Head v8 (Autodesk Fusion 360 design; units mm, degrees)
Autodesk Fusion 360 part; units mm, degrees
note: some values were not read from the file. Set by a fixed rule: which sketch regions a step uses.
sketch "RobotSatan_Outline_2" plane through (0, 0, 0) normal (0, 1, 0) x (1, 0, 0)
  spline S0 degree 3 poles (10.235, 114.5284) (8.6125, 114.5284) (7.297, 113.2125) (7.297, 111.5894) knots 0 0 0 0 1 1 1 1
  spline S1 degree 3 poles (27.2951, 30.5045) (28.9523, 30.5045) (29.7315, 29.3352) (29.7315, 27.8928) knots 0 0 0 0 1 1 1 1
  spline S2 degree 3 poles (10.235, 70.9521) (11.1129, 70.9036) (11.6031, 70.3892) (11.5794, 69.7582) knots 0 0 0 0 1 1 1 1
  spline S3 degree 3 poles (52.0987, 28.374) (53.7202, 28.4279) (55.0356, 29.69) (55.0356, 31.3131) knots 0 0 0 0 1 1 1 1
  spline S4 degree 3 poles (18.5903, 27.8928) (18.5903, 29.3352) (19.3689, 30.5045) (21.0261, 30.5045) knots 0 0 0 0 1 1 1 1
  line L0 (50.7482, 117.3562) -> (50.7482, 115.7102)
  line L1 (7.297, 73.8917) -> (7.297, 82.2427) construction
  line L2 (55.0356, 111.5894) -> (55.0356, 108.6938)
  spline S5 degree 3 poles (11.5794, 115.708) (11.6016, 114.9323) (11.1123, 114.6075) (10.235, 114.5284) knots 0 0 0 0 1 1 1 1
  spline S6 degree 3 poles (11.5794, 19.4245) (11.5794, 17.8014) (12.8944, 16.4854) (14.5168, 16.4854) knots 0 0 0 0 1 1 1 1
  line L3 (27.2951, 23.1855) -> (21.0261, 23.1855)
  spline S7 degree 3 poles (50.7482, 104.5729) (50.749, 105.0607) (51.0594, 105.7079) (52.0987, 105.7553) knots 0 0 0 0 1 1 1 1
  line L4 (29.7315, 27.8928) -> (29.7315, 25.7971)
  line L5 (50.7482, 19.4245) -> (50.7482, 27.1735)
  spline S8 degree 3 poles (50.7482, 117.3562) (50.7482, 118.9793) (49.4332, 120.2947) (47.8108, 120.2947) knots 0 0 0 0 1 1 1 1
  spline S9 degree 3 poles (14.5168, 120.2947) (12.8944, 120.2947) (11.5794, 118.9793) (11.5794, 117.3562) knots 0 0 0 0 1 1 1 1
  line L6 (14.5168, 16.4854) -> (22.8385, 16.4854)
  line L7 (22.3658, 46.6652) -> (19.6342, 46.6652)
  line L8 (28.812, 14.3765) -> (33.4439, 14.3765)
  line L9 (18.5903, 27.8928) -> (18.5903, 25.7971)
  spline S10 degree 3 poles (21.0261, 23.1855) (19.3689, 23.1855) (18.6453, 24.3555) (18.5903, 25.7971) knots 0 0 0 0 1 1 1 1
  spline S11 degree 3 poles (10.235, 28.374) (10.7285, 28.3793) (11.6383, 28.108) (11.5794, 27.2452) knots 0 0 0 0 1 1 1 1
  spline S12 degree 3 poles (11.5794, 43.7193) (11.5828, 43.2312) (11.1144, 42.5873) (10.235, 42.6031) knots 0 0 0 0 1 1 1 1
  spline S13 degree 3 poles (52.0987, 114.5284) (51.2509, 114.5136) (50.7594, 115.2803) (50.7482, 115.7102) knots 0 0 0 0 1 1 1 1
  line L10 (14.5168, 100.5358) -> (47.8108, 100.5358)
  spline S14 degree 3 poles (47.8108, 16.4854) (49.4323, 16.5393) (50.7482, 17.8014) (50.7482, 19.4245) knots 0 0 0 0 1 1 1 1
  line L11 (27.1821, 15.8565) -> (27.1821, 15.6906)
  line L12 (27.2951, 30.5045) -> (21.0261, 30.5045)
  line L13 (61.8594, 0.1406) -> (0.1406, 0.1406)
  line L14 (14.5168, 120.2947) -> (47.8108, 120.2947)
  line L15 (21.0261, 30.5045) -> (27.2951, 30.5045)
  line L16 (21.0261, 23.1855) -> (27.2951, 23.1855)
  spline S15 degree 3 poles (52.0987, 105.7553) (53.7211, 105.7553) (55.0356, 107.0707) (55.0356, 108.6938) knots 0 0 0 0 1 1 1 1
  line L17 (33.4439, 17.1706) -> (28.812, 17.1706)
  spline S16 degree 3 poles (29.7315, 25.7971) (29.7315, 24.3547) (28.9523, 23.1855) (27.2951, 23.1855) knots 0 0 0 0 1 1 1 1
  line L18 (18.5903, 25.7971) -> (18.5903, 27.8928)
  spline S17 degree 3 poles (38.2753, 14.9635) (38.2769, 16.2773) (39.0062, 16.4966) (39.4957, 16.4854) knots 0 0 0 0 1 1 1 1
  spline S18 degree 3 poles (10.235, 42.6031) (8.6125, 42.6031) (7.297, 41.2877) (7.297, 39.6646) knots 0 0 0 0 1 1 1 1
  spline S19 degree 3 poles (10.235, 105.7553) (11.1266, 105.7379) (11.5873, 104.8858) (11.5794, 104.5647) knots 0 0 0 0 1 1 1 1
  line L19 (42.3658, 46.6652) -> (39.6342, 46.6652)
  spline S20 degree 3 poles (35.3373, 12.025) (36.9598, 12.025) (38.2753, 13.3404) (38.2753, 14.9635) knots 0 0 0 0 1 1 1 1
  line L20 (47.8108, 120.2947) -> (14.5168, 120.2947)
  line L21 (39.4957, 16.4854) -> (47.8108, 16.4854)
  line L22 (35.0744, 15.8565) -> (35.0744, 15.6906)
  line L23 (33.4439, 14.3765) -> (28.812, 14.3765)
  line L24 (29.7315, 25.7971) -> (29.7315, 27.8928)
  line L25 (35.0744, 15.6906) -> (35.0744, 15.8565)
  line L26 (7.297, 108.6938) -> (7.297, 111.5894)
  line L27 (11.5794, 115.708) -> (11.5794, 117.3562)
  spline S21 degree 3 poles (27.1821, 15.8565) (27.1821, 16.5823) (27.9117, 17.1706) (28.812, 17.1706) knots 0 0 0 0 1 1 1 1
  line L28 (11.5794, 104.5647) -> (11.5794, 103.4749)
  spline S22 degree 3 poles (50.7482, 69.7345) (50.7292, 70.4446) (51.1934, 70.9205) (52.0987, 70.9521) knots 0 0 0 0 1 1 1 1
  line L29 (7.297, 111.5894) -> (7.297, 108.6938)
  spline S23 degree 3 poles (7.297, 108.6938) (7.3508, 107.0716) (8.6125, 105.7553) (10.235, 105.7553) knots 0 0 0 0 1 1 1 1
  line L30 (11.5794, 117.3562) -> (11.5794, 115.708)
  spline S24 degree 3 poles (55.0356, 111.5894) (55.0356, 113.2125) (53.7211, 114.5284) (52.0987, 114.5284) knots 0 0 0 0 1 1 1 1
  line L31 (50.7482, 104.5729) -> (50.7482, 103.4749)
  line L32 (50.7482, 103.4749) -> (50.7482, 104.5729)
  line L33 (35.3373, 12.025) -> (26.9903, 12.025)
  line L34 (50.7482, 115.7102) -> (50.7482, 117.3562)
  line L35 (11.5794, 69.7582) -> (11.5794, 43.7193)
  line L36 (7.297, 39.6646) -> (7.297, 31.3131)
  line L37 (11.5794, 27.2452) -> (11.5794, 19.4245)
  line L38 (7.297, 31.3131) -> (7.297, 39.6646)
  line L39 (55.0356, 108.6938) -> (55.0356, 111.5894)
  line L40 (50.7482, 27.1735) -> (50.7482, 19.4245)
  line L41 (47.8108, 100.5358) -> (14.5168, 100.5358)
  line L42 (55.0356, 82.2427) -> (55.0356, 73.8917)
  spline S25 degree 3 poles (47.8108, 100.5358) (49.4323, 100.5897) (50.7482, 101.8518) (50.7482, 103.4749) knots 0 0 0 0 1 1 1 1
  line L43 (50.7482, 43.786) -> (50.7482, 69.7345)
  line L44 (28.812, 17.1706) -> (33.4439, 17.1706)
  line L45 (27.1821, 15.6906) -> (27.1821, 15.8565)
  line L46 (11.5794, 103.4749) -> (11.5794, 104.5647)
  line L47 (50.7482, 69.7345) -> (50.7482, 43.786)
  spline S26 degree 3 poles (24.0523, 14.9635) (24.1061, 13.3413) (25.3678, 12.025) (26.9903, 12.025) knots 0 0 0 0 1 1 1 1
  line L48 (11.5794, 43.7193) -> (11.5794, 69.7582)
  spline S27 degree 3 poles (22.8385, 16.4854) (23.3022, 16.5043) (24.0076, 16.1123) (24.0523, 14.9635) knots 0 0 0 0 1 1 1 1
  spline S28 degree 3 poles (35.0744, 15.6906) (35.0744, 14.9648) (34.3442, 14.3765) (33.4439, 14.3765) knots 0 0 0 0 1 1 1 1
  line L49 (26.9903, 12.025) -> (35.3373, 12.025)
  line L50 (55.0356, 73.8917) -> (55.0356, 82.2427)
  line L51 (11.5794, 19.4245) -> (11.5794, 27.2452)
  spline S29 degree 3 poles (7.297, 31.3131) (7.297, 29.69) (8.6125, 28.374) (10.235, 28.374) knots 0 0 0 0 1 1 1 1
  line L52 (32.3658, 46.6652) -> (29.6342, 46.6652)
  line L53 (0.1406, 0.1406) -> (0.1406, 121.8594)
  line L54 (47.8108, 16.4854) -> (39.4957, 16.4854)
  spline S30 degree 3 poles (52.0987, 70.9521) (53.7202, 71.006) (55.0356, 72.2686) (55.0356, 73.8917) knots 0 0 0 0 1 1 1 1
  spline S31 degree 3 poles (33.4439, 17.1706) (34.3442, 17.1706) (35.0744, 16.5823) (35.0744, 15.8565) knots 0 0 0 0 1 1 1 1
  spline S32 degree 3 poles (11.5794, 103.4749) (11.5794, 101.8518) (12.8944, 100.5358) (14.5168, 100.5358) knots 0 0 0 0 1 1 1 1
  line L55 (22.8385, 16.4854) -> (14.5168, 16.4854)
  spline S33 degree 3 poles (55.0356, 39.6646) (55.0356, 41.2877) (53.7211, 42.6031) (52.0987, 42.6031) knots 0 0 0 0 1 1 1 1
  spline S34 degree 3 poles (50.7482, 27.1735) (50.7463, 28.0057) (51.624, 28.3964) (52.0987, 28.374) knots 0 0 0 0 1 1 1 1
  spline S35 degree 3 poles (7.297, 73.8917) (7.297, 72.2686) (8.6125, 70.9521) (10.235, 70.9521) knots 0 0 0 0 1 1 1 1
  line L56 (55.0356, 31.3131) -> (55.0356, 39.6646)
  spline S36 degree 3 poles (28.812, 14.3765) (27.9117, 14.3765) (27.212, 14.9652) (27.1821, 15.6906) knots 0 0 0 0 1 1 1 1
  spline S37 degree 3 poles (52.0987, 42.6031) (51.0209, 42.5992) (50.737, 43.4395) (50.7482, 43.786) knots 0 0 0 0 1 1 1 1
  line L57 (55.0356, 39.6646) -> (55.0356, 31.3131)
  line L58 (61.8594, 121.8594) -> (61.8594, 0.1406)
  line L59 (0.1406, 121.8594) -> (61.8594, 121.8594)
  spline S38 degree 3 poles (32.4655, 143.4) (23.7353, 143.4503) (14.7543, 139.3652) (8.8222, 129.236) knots 0 0 0 0 1 1 1 1
  spline S39 degree 3 poles (-8.0125, 95.4824) (-4.6273, 94.9818) (-1.6894, 95.1386) (0.7276, 95.7376) knots 0 0 0 0 1 1 1 1
  spline S40 degree 3 poles (3.7466, 109.0725) (3.7475, 109.0731) (3.7485, 109.0742) (3.7494, 109.0748) knots 0 0 0 0 1 1 1 1
  spline S41 degree 3 poles (61.918, 105.4461) (62.3441, 106.388) (61.5048, 105.6412) (58.7789, 105.6098) knots 0 0 0 0 1 1 1 1
  spline S42 degree 3 poles (8.8222, 129.236) (6.0519, 124.5056) (6.9924, 118.038) (5.4372, 112.5441) knots 0 0 0 0 1 1 1 1
  spline S43 degree 3 poles (53.6696, 133.8916) (48.6461, 139.6563) (40.6666, 143.3529) (32.4655, 143.4001) knots 0 0 0 0 1 1 1 1
  spline S44 degree 3 poles (24.2524, 66.9983) (22.9484, 63.6454) (80.6805, 92.1452) (55.5432, 101.6168) knots 0 0 0 0 1 1 1 1
  spline S45 degree 3 poles (3.5267, 109.1834) (2.9555, 109.457) (1.8977, 109.5026) (0.8037, 109.1696) knots 0 0 0 0 1 1 1 1
  spline S46 degree 3 poles (5.4372, 112.5441) (5.2254, 110.4206) (4.1381, 109.3015) (3.7494, 109.0747) knots 0 0 0 0 1 1 1 1
  spline S47 degree 3 poles (3.6435, 109.1249) (3.6041, 109.1443) (3.5666, 109.1642) (3.5267, 109.1834) knots 0 0 0 0 1 1 1 1
  spline S48 degree 3 poles (3.7615, 109.0654) (3.7566, 109.0679) (3.7515, 109.0701) (3.7466, 109.0725) knots 0 0 0 0 1 1 1 1
  line L60 (32.4655, 143.4) -> (32.4655, 143.4001)
  spline S49 degree 3 poles (0.7276, 95.7376) (-16.7215, 76.039) (36.655, 80.3237) (24.2524, 66.9983) knots 0 0 0 0 1 1 1 1
  spline S50 degree 3 poles (58.7789, 105.6098) (59.7712, 116.9489) (58.3276, 128.5464) (53.6696, 133.8916) knots 0 0 0 0 1 1 1 1
  spline S51 degree 3 poles (55.5432, 101.6168) (57.9111, 102.4984) (60.0987, 103.7515) (61.918, 105.4461) knots 0 0 0 0 1 1 1 1
  spline S52 degree 3 poles (3.6562, 109.1475) (3.6494, 109.1382) (3.6488, 109.1332) (3.6435, 109.1249) knots 0 0 0 0 1 1 1 1
  line L61 (32.4655, 143.4001) -> (32.4655, 143.4)
  spline S53 degree 3 poles (3.7494, 109.0748) (3.7206, 109.096) (3.6836, 109.1282) (3.6562, 109.1475) knots 0 0 0 0 1 1 1 1
  spline S54 degree 3 poles (3.7494, 109.0747) (3.7531, 109.0719) (3.7577, 109.0682) (3.7615, 109.0654) knots 0 0 0 0 1 1 1 1
  spline S55 degree 3 poles (0.8037, 109.1696) (-12.8378, 101.9111) (5.3858, 99.0443) (-8.0125, 95.4824) knots 0 0 0 0 1 1 1 1
  line L62 (7.147, 111.5894) -> (7.147, 108.6913)
  spline S56 degree 3 poles (7.147, 108.6913) (7.147, 108.6905) (7.1471, 108.6897) (7.1471, 108.6888) (7.2034, 106.9921) (8.5306, 105.6061) (10.2335, 105.6053) knots -0.000511 -0.000511 -0.000511 -0.000511 0 0 0 0.999702 0.999702 0.999702 0.999702
  spline S57 degree 3 poles (10.2335, 105.6053) (10.7603, 105.5944) (11.1167, 105.257) (11.2985, 104.9443) (11.3914, 104.7845) (11.4309, 104.6263) (11.4294, 104.5684) (11.4294, 104.5677) (11.4294, 104.5671) (11.4294, 104.5665) knots 0.000588 0.000588 0.000588 0.000588 0.661876 0.661876 0.661876 1 1 1 1.001915 1.001915 1.001915 1.001915
  line L63 (11.4294, 103.4749) -> (11.4294, 104.5665)
  spline S58 degree 3 poles (11.4294, 103.4749) (11.4294, 101.7707) (12.8133, 100.3858) (14.5168, 100.3858) knots 0 0 0 0 1 1 1 1
  line L64 (14.5168, 100.3858) -> (47.8133, 100.3858)
  spline S59 degree 3 poles (47.8133, 100.3858) (47.8141, 100.3859) (47.8149, 100.3859) (47.8158, 100.3859) (49.5123, 100.4423) (50.8982, 101.7707) (50.8982, 103.4749) knots -0.000512 -0.000512 -0.000512 -0.000512 0 0 0 1 1 1 1
  line L65 (50.8982, 103.4749) -> (50.8982, 104.5727)
  spline S60 degree 3 poles (50.8982, 104.5727) (50.8988, 104.9717) (51.1034, 105.4899) (51.9385, 105.5917) (51.9905, 105.598) (52.045, 105.6026) (52.1022, 105.6053) knots 0 0 0 0 0.940352 0.940352 0.940352 0.998867 0.998867 0.998867 0.998867
  spline S61 degree 3 poles (52.1022, 105.6053) (53.8041, 105.6072) (55.1856, 106.9909) (55.1856, 108.6938) knots 0.000688 0.000688 0.000688 0.000688 1 1 1 1
  line L66 (55.1856, 108.6938) -> (55.1856, 111.5894)
  spline S62 degree 3 poles (55.1856, 111.5894) (55.1856, 113.2935) (53.8022, 114.6784) (52.0987, 114.6784) (52.0982, 114.6784) (52.0978, 114.6784) (52.0974, 114.6784) knots 0 0 0 0 1 1 1 1.00027 1.00027 1.00027 1.00027
  spline S63 degree 3 poles (52.0974, 114.6784) (52.0969, 114.6784) (52.0965, 114.6784) (52.096, 114.6784) (51.4522, 114.6671) (51.039, 115.1733) (50.9284, 115.5426) (50.9093, 115.6064) (50.8996, 115.665) (50.8982, 115.7123) knots -0.000517 -0.000517 -0.000517 -0.000517 0 0 0 0.851167 0.851167 0.851167 0.998126 0.998126 0.998126 0.998126
  line L67 (50.8982, 115.7123) -> (50.8982, 117.3562)
  spline S64 degree 3 poles (50.8982, 117.3562) (50.8982, 119.0603) (49.5143, 120.4447) (47.8108, 120.4447) knots 0 0 0 0 1 1 1 1
  line L68 (47.8108, 120.4447) -> (14.5168, 120.4447)
  spline S65 degree 3 poles (14.5168, 120.4447) (12.8133, 120.4447) (11.4294, 119.0603) (11.4294, 117.3562) knots 0 0 0 0 1 1 1 1
  line L69 (11.4294, 117.3562) -> (11.4294, 115.7059)
  spline S66 degree 3 poles (11.4294, 115.7059) (11.4294, 115.7052) (11.4294, 115.7045) (11.4295, 115.7037) (11.4442, 115.1885) (11.2516, 114.9477) (10.82, 114.7957) (10.6572, 114.7384) (10.4586, 114.6996) (10.2281, 114.6784) knots -0.000923 -0.000923 -0.000923 -0.000923 0 0 0 0.724154 0.724154 0.724154 0.997406 0.997406 0.997406 0.997406
  spline S67 degree 3 poles (10.2281, 114.6784) (8.5277, 114.6747) (7.147, 113.2913) (7.147, 111.5894) knots 0.001348 0.001348 0.001348 0.001348 1 1 1 1
  line L70 (6.147, 108.6747) -> (6.147, 111.5894)
  spline S68 degree 3 poles (10.1748, 115.678) (8.283, 115.6506) (6.6845, 114.3247) (6.2588, 112.5418) (6.1856, 112.2353) (6.147, 111.9157) (6.147, 111.5894) knots 0.008942 0.008942 0.008942 0.008942 0.854617 0.854617 0.854617 1 1 1 1
  spline S69 degree 3 poles (10.4294, 115.7213) (10.3703, 115.7058) (10.2833, 115.6894) (10.1748, 115.678) knots 0.796356 0.796356 0.796356 0.796356 0.976812 0.976812 0.976812 0.976812
  line L71 (10.4294, 115.7213) -> (10.4294, 117.3562)
  spline S70 degree 3 poles (14.5168, 121.4447) (12.6021, 121.4447) (10.9764, 120.1145) (10.5432, 118.3172) (10.4687, 118.0081) (10.4294, 117.6855) (10.4294, 117.3562) knots 0 0 0 0 0.85324 0.85324 0.85324 1 1 1 1
  line L72 (14.5168, 121.4447) -> (47.8108, 121.4447)
  spline S71 degree 3 poles (51.8982, 117.3562) (51.8982, 119.2711) (50.5687, 120.8973) (48.7717, 121.3308) (48.4626, 121.4054) (48.1401, 121.4447) (47.8108, 121.4447) knots 0 0 0 0 0.853239 0.853239 0.853239 1 1 1 1
  line L73 (51.8982, 115.806) -> (51.8982, 117.3562)
  spline S72 degree 3 poles (52.0886, 115.6784) (52.0852, 115.6784) (52.0819, 115.6783) (52.0785, 115.6783) (52.0071, 115.677) (51.9994, 115.6875) (51.9497, 115.738) (51.9295, 115.7586) (51.9098, 115.7856) (51.8982, 115.806) knots -0.003967 -0.003967 -0.003967 -0.003967 0 0 0 0.485877 0.485877 0.485877 0.683858 0.683858 0.683858 0.683858
  spline S73 degree 3 poles (56.1856, 111.5894) (56.1856, 113.504) (54.8569, 115.1307) (53.0598, 115.5645) (52.7507, 115.6391) (52.4281, 115.6784) (52.0987, 115.6784) (52.0953, 115.6784) (52.092, 115.6784) (52.0886, 115.6784) knots 0 0 0 0 0.853226 0.853226 0.853226 1 1 1 1.002073 1.002073 1.002073 1.002073
  line L74 (56.1856, 111.5894) -> (56.1856, 108.6938)
  spline S74 degree 3 poles (52.1309, 104.6054) (54.03, 104.6202) (55.6386, 105.9437) (56.0708, 107.7285) (56.1459, 108.0389) (56.1856, 108.3629) (56.1856, 108.6938) knots 0.004787 0.004787 0.004787 0.004787 0.852555 0.852555 0.852555 1 1 1 1
  spline S75 degree 3 poles (51.8982, 104.5603) (51.9279, 104.5736) (51.9958, 104.5973) (52.1309, 104.6054) knots 0.740647 0.740647 0.740647 0.740647 0.987986 0.987986 0.987986 0.987986
  line L75 (51.8982, 104.5603) -> (51.8982, 103.4749)
  spline S76 degree 3 poles (47.8299, 99.3858) (47.8362, 99.386) (47.8426, 99.3863) (47.849, 99.3865) (49.5971, 99.4445) (51.1264, 100.5496) (51.6797, 102.1591) (51.8217, 102.5721) (51.8982, 103.0166) (51.8982, 103.4749) knots -0.003923 -0.003923 -0.003923 -0.003923 0 0 0 0.795824 0.795824 0.795824 1 1 1 1
  line L76 (47.8299, 99.3858) -> (14.5168, 99.3858)
  spline S77 degree 3 poles (10.4294, 103.4749) (10.4294, 101.5585) (11.7608, 99.9309) (13.56, 99.4987) (13.8678, 99.4248) (14.189, 99.3858) (14.5168, 99.3858) knots 0 0 0 0 0.853916 0.853916 0.853916 1 1 1 1
  line L77 (10.4294, 104.4494) -> (10.4294, 103.4749)
  spline S78 degree 3 poles (10.2185, 104.6053) (10.2902, 104.6022) (10.3098, 104.5874) (10.3672, 104.529) (10.3908, 104.505) (10.4139, 104.4747) (10.4294, 104.4494) knots 0.01242 0.01242 0.01242 0.01242 0.459325 0.459325 0.459325 0.642978 0.642978 0.642978 0.642978
  spline S79 degree 3 poles (6.147, 108.6747) (6.1472, 108.6684) (6.1474, 108.662) (6.1476, 108.6557) (6.2056, 106.9088) (7.308, 105.3803) (8.9151, 104.8253) (9.3242, 104.6841) (9.7645, 104.6071) (10.2185, 104.6053) knots -0.003918 -0.003918 -0.003918 -0.003918 0 0 0 0.795118 0.795118 0.795118 0.997552 0.997552 0.997552 0.997552
  line L78 (10.4294, 115.7213) -> (51.8982, 115.806)
  line L79 (52.1309, 104.6054) -> (10.2185, 104.6053)
  dimension "d3" = 0.15
  dimension "d4" = 1.15
  measures "d3" distance of L29
  measures "d4" distance of L26
extrude "Extrude1" add sketch "RobotSatan_Outline_2" along normal blind 3 contours S0 L0 L2 S5 S7 S13 S15 S19 L26 L27 L29 S23 L30 S24 L34 L39 L78 L79 | S0 S5 S19 L26 L27 L29 S23 L30 L62 S56 S57 L69 S66 S67 L78 L79 | L0 S8 S9 L14 L20 L27 L30 L34 L67 S64 L68 S65 L69 L78 | L0 S8 S9 L14 L20 L27 L30 L34 L78 | L67 S64 L68 S65 L69 L71 S70 L72 S71 L73 L78 | L62 S56 S57 L69 S66 S67 L70 S68 S69 S79 L78 L79 | L0 L2 S7 S13 S15 S24 L34 L39 S60 S61 L66 S62 S63 L67 L78 L79 | S7 L10 S19 L28 L31 L32 L41 S25 L46 S32 L79 | S7 L10 S19 L28 L31 L32 L41 S25 L46 S32 S57 L63 S58 L64 S59 L65 S60 L79 | S60 S61 L66 S62 S63 L67 S72 S73 L74 S74 L78 L79 | S57 L63 S58 L64 S59 L65 S60 S75 L75 S76 L76 S77 L77 S78 L79 | L53 L58 L59 S39 S41 S42 S44 S45 S46 S47 S49 S50 S51 S52 S53 S55 | L53 S49 | L53 S39 S55 | L59 S38 S42 S43 S50 makes body 1
extrude "Extrude2" add sketch "RobotSatan_Outline_2" against normal blind 5 separate body contours L62 S56 S57 L69 S66 S67 L70 S68 S69 S79 L78 L79 | S60 S61 L66 S62 S63 L67 S72 S73 L74 S74 L78 L79 makes body 2 at (6.2362, -2.8704, -107.9159) makes body 3 at (54.3636, -2.2222, -114.992)
extrude "Extrude3" cut sketch "RobotSatan_Outline_2" along normal through all contours S0 L0 L2 S5 S7 S13 S15 S19 L26 L27 L29 S23 L30 S24 L34 L39 L78 L79 bodies 1
sketch "Sketch3" plane through (0, 0, 0) normal (0, -1, 0) x (1, 0, 0)
  line L0 (11.5781, -104.6053) -> (50.7487, -104.6054)
  spline S0 degree 3 poles (50.7487, -104.6054) (50.763, -105.089) (51.0823, -105.7089) (52.0987, -105.7553) knots 0.022041 0.022041 0.022041 0.022041 1 1 1 1
  spline S1 degree 3 poles (52.0987, -105.7553) (53.7211, -105.7553) (55.0356, -107.0707) (55.0356, -108.6938) knots 0 0 0 0 1 1 1 1
  line L1 (55.0356, -108.6938) -> (55.0356, -111.5894)
  spline S2 degree 3 poles (55.0356, -111.5894) (55.0356, -113.2125) (53.7211, -114.5284) (52.0987, -114.5284) knots 0 0 0 0 1 1 1 1
  spline S3 degree 3 poles (52.0987, -114.5284) (51.2509, -114.5136) (50.7594, -115.2803) (50.7482, -115.7102) knots 0 0 0 0 1 1 1 1
  line L2 (50.7482, -115.7102) -> (50.7482, -115.8036)
  line L3 (50.7482, -115.8036) -> (11.5794, -115.7236)
  line L4 (11.5794, -115.7236) -> (11.5794, -115.708)
  spline S4 degree 3 poles (11.5794, -115.708) (11.6016, -114.9323) (11.1123, -114.6075) (10.235, -114.5284) knots 0 0 0 0 1 1 1 1
  spline S5 degree 3 poles (10.235, -114.5284) (8.6125, -114.5284) (7.297, -113.2125) (7.297, -111.5894) knots 0 0 0 0 1 1 1 1
  line L5 (7.297, -111.5894) -> (7.297, -108.6938)
  spline S6 degree 3 poles (7.297, -108.6938) (7.3508, -107.0716) (8.6125, -105.7553) (10.235, -105.7553) knots 0 0 0 0 1 1 1 1
  spline S7 degree 3 poles (10.235, -105.7553) (11.0912, -105.7386) (11.55, -104.9521) (11.5781, -104.6053) knots 0 0 0 0 0.96031 0.96031 0.96031 0.96031
  spline S8 degree 3 poles (61.8594, -105.9188) (61.4992, -105.9443) (60.5269, -105.63) (58.7789, -105.6098) knots 0.358724 0.358724 0.358724 0.358724 1 1 1 1
  line L6 (61.8594, -105.9188) -> (61.8594, -105.3918)
  spline S9 degree 3 poles (55.5432, -101.6168) (57.8857, -102.489) (60.0518, -103.7247) (61.8594, -105.3918) knots 0 0 0 0 0.989277 0.989277 0.989277 0.989277
  spline S10 degree 3 poles (61.8594, -95.5661) (61.6019, -97.9517) (59.7123, -100.046) (55.5432, -101.6168) knots 0.834148 0.834148 0.834148 0.834148 1 1 1 1
  line L7 (61.8594, -95.5661) -> (61.8594, -94.3906)
  spline S11 degree 3 poles (24.2524, -66.9983) (23.1996, -64.2912) (60.6331, -82.3492) (61.8594, -94.3906) knots 0 0 0 0 0.807411 0.807411 0.807411 0.807411
  spline S12 degree 3 poles (0.7276, -95.7376) (-16.7215, -76.039) (36.655, -80.3237) (24.2524, -66.9983) knots 0 0 0 0 1 1 1 1
  spline S13 degree 3 poles (-8.0125, -95.4824) (-4.6273, -94.9818) (-1.6894, -95.1386) (0.7276, -95.7376) knots 0 0 0 0 1 1 1 1
  spline S14 degree 3 poles (0.8037, -109.1696) (-12.8378, -101.9111) (5.3858, -99.0443) (-8.0125, -95.4824) knots 0 0 0 0 1 1 1 1
  spline S15 degree 3 poles (3.5267, -109.1834) (2.9555, -109.457) (1.8977, -109.5026) (0.8037, -109.1696) knots 0 0 0 0 1 1 1 1
  spline S16 degree 3 poles (3.6435, -109.1249) (3.6041, -109.1443) (3.5666, -109.1642) (3.5267, -109.1834) knots 0 0 0 0 1 1 1 1
  spline S17 degree 3 poles (3.6562, -109.1475) (3.6494, -109.1382) (3.6488, -109.1332) (3.6435, -109.1249) knots 0 0 0 0 1 1 1 1
  spline S18 degree 3 poles (3.7494, -109.0748) (3.7206, -109.096) (3.6836, -109.1282) (3.6562, -109.1475) knots 0 0 0 0 1 1 1 1
  spline S19 degree 3 poles (3.7466, -109.0725) (3.7475, -109.0731) (3.7485, -109.0742) (3.7494, -109.0748) knots 0 0 0 0 1 1 1 1
  spline S20 degree 3 poles (3.7615, -109.0654) (3.7566, -109.0679) (3.7515, -109.0701) (3.7466, -109.0725) knots 0 0 0 0 1 1 1 1
  spline S21 degree 3 poles (3.7494, -109.0747) (3.7531, -109.0719) (3.7577, -109.0682) (3.7615, -109.0654) knots 0 0 0 0 1 1 1 1
  spline S22 degree 3 poles (5.4372, -112.5441) (5.2254, -110.4206) (4.1381, -109.3015) (3.7494, -109.0747) knots 0 0 0 0 1 1 1 1
  spline S23 degree 3 poles (8.8222, -129.236) (6.0519, -124.5056) (6.9924, -118.038) (5.4372, -112.5441) knots 0 0 0 0 1 1 1 1
  spline S24 degree 3 poles (32.4655, -143.4) (23.7353, -143.4503) (14.7543, -139.3652) (8.8222, -129.236) knots 0 0 0 0 1 1 1 1
  line L8 (32.4655, -143.4) -> (32.4655, -143.4001)
  spline S25 degree 3 poles (53.6696, -133.8916) (48.6461, -139.6563) (40.6666, -143.3529) (32.4655, -143.4001) knots 0 0 0 0 1 1 1 1
  spline S26 degree 3 poles (58.7789, -105.6098) (59.7712, -116.9489) (58.3276, -128.5464) (53.6696, -133.8916) knots 0 0 0 0 1 1 1 1
  line L9 (31.1979, -84.3033) -> (31.1322, -116.4684) construction
  line L10 (14.5168, -100.3858) -> (47.8133, -100.3858)
  line L11 (-12, -104) -> (70.3181, -104.0002) construction
  circle A0 centre (6.1576, -104) radius 1.5
  circle A1 centre (56.1577, -104.0013) radius 1.5
  dimension "d10" = 3
  dimension "d11" = 25
  dimension "d12" = 3
  dimension "d13" = 25
  constraint perpendicular L3 L9
  constraint midpoint L9 L10
  constraint parallel L0 L11
  constraint coincident L11
  measures "d10" diameter of A0
  measures "d12" diameter of A1
extrude "Extrude4" add sketch "Sketch3" along normal blind 11 contours A0 | A1 bodies 1
